Autodesk Inventor part; units mm, degrees
(part 2 of 2)
  line L515 (266.104, 188.0456) -> (266.9242, 187.2258) construction
  line L516 (266.9242, 187.2258) -> (266.9242, 186.2158) construction
  line L517 (266.9242, 186.2158) -> (266.9242, 185.2058) construction
  line L518 (266.9242, 185.2058) -> (266.104, 184.3855) construction
  line L519 (266.104, 184.3855) -> (265.094, 184.3855) construction
  spline S46 degree 3 poles (265.094, 168.3853) (264.084, 168.3853) (263.2642, 169.2052) (263.2642, 170.2152) (263.2642, 171.2255) (264.084, 172.0454) (265.094, 172.0454) (266.104, 172.0454) (266.9242, 171.2255) (266.9242, 170.2152) (266.9242, 169.2052) (266.104, 168.3853) (265.094, 168.3853) knots 0 0 0 0 1 1 1 2 2 2 3 3 3 4 4 4 4
  line L520 (265.094, 168.3853) -> (264.084, 168.3853) construction
  line L521 (264.084, 168.3853) -> (263.2642, 169.2052) construction
  line L522 (263.2642, 169.2052) -> (263.2642, 170.2152) construction
  line L523 (263.2642, 170.2152) -> (263.2642, 171.2255) construction
  line L524 (263.2642, 171.2255) -> (264.084, 172.0454) construction
  line L525 (264.084, 172.0454) -> (265.094, 172.0454) construction
  line L526 (265.094, 172.0454) -> (266.104, 172.0454) construction
  line L527 (266.104, 172.0454) -> (266.9242, 171.2255) construction
  line L528 (266.9242, 171.2255) -> (266.9242, 170.2152) construction
  line L529 (266.9242, 170.2152) -> (266.9242, 169.2052) construction
  line L530 (266.9242, 169.2052) -> (266.104, 168.3853) construction
  line L531 (266.104, 168.3853) -> (265.094, 168.3853) construction
  spline S47 degree 3 poles (265.0305, 152.3834) (264.0262, 152.3834) (263.2102, 153.2036) (263.2102, 154.2136) (263.2102, 155.2236) (264.0262, 156.0434) (265.0305, 156.0434) (266.0366, 156.0434) (266.8526, 155.2236) (266.8526, 154.2136) (266.8526, 153.2036) (266.0366, 152.3834) (265.0305, 152.3834) knots 0 0 0 0 1 1 1 2 2 2 3 3 3 4 4 4 4
  line L532 (265.0305, 152.3834) -> (264.0262, 152.3834) construction
  line L533 (264.0262, 152.3834) -> (263.2102, 153.2036) construction
  line L534 (263.2102, 153.2036) -> (263.2102, 154.2136) construction
  line L535 (263.2102, 154.2136) -> (263.2102, 155.2236) construction
  line L536 (263.2102, 155.2236) -> (264.0262, 156.0434) construction
  line L537 (264.0262, 156.0434) -> (265.0305, 156.0434) construction
  line L538 (265.0305, 156.0434) -> (266.0366, 156.0434) construction
  line L539 (266.0366, 156.0434) -> (266.8526, 155.2236) construction
  line L540 (266.8526, 155.2236) -> (266.8526, 154.2136) construction
  line L541 (266.8526, 154.2136) -> (266.8526, 153.2036) construction
  line L542 (266.8526, 153.2036) -> (266.0366, 152.3834) construction
  line L543 (266.0366, 152.3834) -> (265.0305, 152.3834) construction
  spline S48 degree 3 poles (265.0305, 136.3832) (264.0262, 136.3832) (263.2102, 137.203) (263.2102, 138.213) (263.2102, 139.2234) (264.0262, 140.0432) (265.0305, 140.0432) (266.0366, 140.0432) (266.8526, 139.2234) (266.8526, 138.213) (266.8526, 137.203) (266.0366, 136.3832) (265.0305, 136.3832) knots 0 0 0 0 1 1 1 2 2 2 3 3 3 4 4 4 4
  line L544 (265.0305, 136.3832) -> (264.0262, 136.3832) construction
  line L545 (264.0262, 136.3832) -> (263.2102, 137.203) construction
  line L546 (263.2102, 137.203) -> (263.2102, 138.213) construction
  line L547 (263.2102, 138.213) -> (263.2102, 139.2234) construction
  line L548 (263.2102, 139.2234) -> (264.0262, 140.0432) construction
  line L549 (264.0262, 140.0432) -> (265.0305, 140.0432) construction
  line L550 (265.0305, 140.0432) -> (266.0366, 140.0432) construction
  line L551 (266.0366, 140.0432) -> (266.8526, 139.2234) construction
  line L552 (266.8526, 139.2234) -> (266.8526, 138.213) construction
  line L553 (266.8526, 138.213) -> (266.8526, 137.203) construction
  line L554 (266.8526, 137.203) -> (266.0366, 136.3832) construction
  line L555 (266.0366, 136.3832) -> (265.0305, 136.3832) construction
  spline S49 degree 3 poles (264.901, 120.384) (263.9062, 120.384) (263.0987, 121.2039) (263.0987, 122.2142) (263.0987, 123.2228) (263.9062, 124.0427) (264.901, 124.0427) (265.8962, 124.0427) (266.7037, 123.2228) (266.7037, 122.2142) (266.7037, 121.2039) (265.8962, 120.384) (264.901, 120.384) knots 0 0 0 0 1 1 1 2 2 2 3 3 3 4 4 4 4
  line L556 (264.901, 120.384) -> (263.9062, 120.384) construction
  line L557 (263.9062, 120.384) -> (263.0987, 121.2039) construction
  line L558 (263.0987, 121.2039) -> (263.0987, 122.2142) construction
  line L559 (263.0987, 122.2142) -> (263.0987, 123.2228) construction
  line L560 (263.0987, 123.2228) -> (263.9062, 124.0427) construction
  line L561 (263.9062, 124.0427) -> (264.901, 124.0427) construction
  line L562 (264.901, 124.0427) -> (265.8962, 124.0427) construction
  line L563 (265.8962, 124.0427) -> (266.7037, 123.2228) construction
  line L564 (266.7037, 123.2228) -> (266.7037, 122.2142) construction
  line L565 (266.7037, 122.2142) -> (266.7037, 121.2039) construction
  line L566 (266.7037, 121.2039) -> (265.8962, 120.384) construction
  line L567 (265.8962, 120.384) -> (264.901, 120.384) construction
  spline S50 degree 3 poles (282.3572, 87.3704) (282.3572, 88.3808) (283.1771, 89.2007) (284.1871, 89.2007) (285.1974, 89.2007) (286.0173, 88.3808) (286.0173, 87.3704) (286.0173, 86.3604) (285.1974, 85.5406) (284.1871, 85.5406) (283.1771, 85.5406) (282.3572, 86.3604) (282.3572, 87.3704) knots 0 0 0 0 1 1 1 2 2 2 3 3 3 4 4 4 4
  line L568 (282.3572, 87.3704) -> (282.3572, 88.3808) construction
  line L569 (282.3572, 88.3808) -> (283.1771, 89.2007) construction
  line L570 (283.1771, 89.2007) -> (284.1871, 89.2007) construction
  line L571 (284.1871, 89.2007) -> (285.1974, 89.2007) construction
  line L572 (285.1974, 89.2007) -> (286.0173, 88.3808) construction
  line L573 (286.0173, 88.3808) -> (286.0173, 87.3704) construction
  line L574 (286.0173, 87.3704) -> (286.0173, 86.3604) construction
  line L575 (286.0173, 86.3604) -> (285.1974, 85.5406) construction
  line L576 (285.1974, 85.5406) -> (284.1871, 85.5406) construction
  line L577 (284.1871, 85.5406) -> (283.1771, 85.5406) construction
  line L578 (283.1771, 85.5406) -> (282.3572, 86.3604) construction
  line L579 (282.3572, 86.3604) -> (282.3572, 87.3704) construction
  spline S51 degree 3 poles (266.3566, 87.3704) (266.3566, 88.3808) (267.1768, 89.2007) (268.1868, 89.2007) (269.1968, 89.2007) (270.0167, 88.3808) (270.0167, 87.3704) (270.0167, 86.3604) (269.1968, 85.5406) (268.1868, 85.5406) (267.1768, 85.5406) (266.3566, 86.3604) (266.3566, 87.3704) knots 0 0 0 0 1 1 1 2 2 2 3 3 3 4 4 4 4
  line L580 (266.3566, 87.3704) -> (266.3566, 88.3808) construction
  line L581 (266.3566, 88.3808) -> (267.1768, 89.2007) construction
  line L582 (267.1768, 89.2007) -> (268.1868, 89.2007) construction
  line L583 (268.1868, 89.2007) -> (269.1968, 89.2007) construction
  line L584 (269.1968, 89.2007) -> (270.0167, 88.3808) construction
  line L585 (270.0167, 88.3808) -> (270.0167, 87.3704) construction
  line L586 (270.0167, 87.3704) -> (270.0167, 86.3604) construction
  line L587 (270.0167, 86.3604) -> (269.1968, 85.5406) construction
  line L588 (269.1968, 85.5406) -> (268.1868, 85.5406) construction
  line L589 (268.1868, 85.5406) -> (267.1768, 85.5406) construction
  line L590 (267.1768, 85.5406) -> (266.3566, 86.3604) construction
  line L591 (266.3566, 86.3604) -> (266.3566, 87.3704) construction
  spline S52 degree 3 poles (254.015, 87.4339) (254.015, 88.4387) (253.1952, 89.2543) (252.1852, 89.2543) (251.1748, 89.2543) (250.355, 88.4387) (250.355, 87.4339) (250.355, 86.4292) (251.1748, 85.6122) (252.1852, 85.6122) (253.1952, 85.6122) (254.015, 86.4292) (254.015, 87.4339) knots 0 0 0 0 1 1 1 2 2 2 3 3 3 4 4 4 4
  line L592 (254.015, 87.4339) -> (254.015, 88.4387) construction
  line L593 (254.015, 88.4387) -> (253.1952, 89.2543) construction
  line L594 (253.1952, 89.2543) -> (252.1852, 89.2543) construction
  line L595 (252.1852, 89.2543) -> (251.1748, 89.2543) construction
  line L596 (251.1748, 89.2543) -> (250.355, 88.4387) construction
  line L597 (250.355, 88.4387) -> (250.355, 87.4339) construction
  line L598 (250.355, 87.4339) -> (250.355, 86.4292) construction
  line L599 (250.355, 86.4292) -> (251.1748, 85.6122) construction
  line L600 (251.1748, 85.6122) -> (252.1852, 85.6122) construction
  line L601 (252.1852, 85.6122) -> (253.1952, 85.6122) construction
  line L602 (253.1952, 85.6122) -> (254.015, 86.4292) construction
  line L603 (254.015, 86.4292) -> (254.015, 87.4339) construction
  spline S53 degree 3 poles (234.3547, 87.4339) (234.3547, 88.4387) (235.1746, 89.2543) (236.1846, 89.2543) (237.1946, 89.2543) (238.0148, 88.4387) (238.0148, 87.4339) (238.0148, 86.4292) (237.1946, 85.6122) (236.1846, 85.6122) (235.1746, 85.6122) (234.3547, 86.4292) (234.3547, 87.4339) knots 0 0 0 0 1 1 1 2 2 2 3 3 3 4 4 4 4
  line L604 (234.3547, 87.4339) -> (234.3547, 88.4387) construction
  line L605 (234.3547, 88.4387) -> (235.1746, 89.2543) construction
  line L606 (235.1746, 89.2543) -> (236.1846, 89.2543) construction
  line L607 (236.1846, 89.2543) -> (237.1946, 89.2543) construction
  line L608 (237.1946, 89.2543) -> (238.0148, 88.4387) construction
  line L609 (238.0148, 88.4387) -> (238.0148, 87.4339) construction
  line L610 (238.0148, 87.4339) -> (238.0148, 86.4292) construction
  line L611 (238.0148, 86.4292) -> (237.1946, 85.6122) construction
  line L612 (237.1946, 85.6122) -> (236.1846, 85.6122) construction
  line L613 (236.1846, 85.6122) -> (235.1746, 85.6122) construction
  line L614 (235.1746, 85.6122) -> (234.3547, 86.4292) construction
  line L615 (234.3547, 86.4292) -> (234.3547, 87.4339) construction
  spline S54 degree 3 poles (218.3542, 87.5634) (218.3542, 88.5586) (219.1754, 89.3661) (220.1844, 89.3661) (221.1944, 89.3661) (222.0142, 88.5586) (222.0142, 87.5634) (222.0142, 86.5686) (221.1944, 85.7611) (220.1844, 85.7611) (219.1754, 85.7611) (218.3542, 86.5686) (218.3542, 87.5634) knots 0 0 0 0 1 1 1 2 2 2 3 3 3 4 4 4 4
  line L616 (218.3542, 87.5634) -> (218.3542, 88.5586) construction
  line L617 (218.3542, 88.5586) -> (219.1754, 89.3661) construction
  line L618 (219.1754, 89.3661) -> (220.1844, 89.3661) construction
  line L619 (220.1844, 89.3661) -> (221.1944, 89.3661) construction
  line L620 (221.1944, 89.3661) -> (222.0142, 88.5586) construction
  line L621 (222.0142, 88.5586) -> (222.0142, 87.5634) construction
  line L622 (222.0142, 87.5634) -> (222.0142, 86.5686) construction
  line L623 (222.0142, 86.5686) -> (221.1944, 85.7611) construction
  line L624 (221.1944, 85.7611) -> (220.1844, 85.7611) construction
  line L625 (220.1844, 85.7611) -> (219.1754, 85.7611) construction
  line L626 (219.1754, 85.7611) -> (218.3542, 86.5686) construction
  line L627 (218.3542, 86.5686) -> (218.3542, 87.5634) construction
  spline S55 degree 3 poles (282.3569, 7.3714) (282.3569, 8.3814) (283.1771, 9.2012) (284.1871, 9.2012) (285.1971, 9.2012) (286.0169, 8.3814) (286.0169, 7.3714) (286.0169, 6.3614) (285.1971, 5.5412) (284.1871, 5.5412) (283.1771, 5.5412) (282.3569, 6.3614) (282.3569, 7.3714) knots 0 0 0 0 1 1 1 2 2 2 3 3 3 4 4 4 4
  line L628 (282.3569, 7.3714) -> (282.3569, 8.3814) construction
  line L629 (282.3569, 8.3814) -> (283.1771, 9.2012) construction
  line L630 (283.1771, 9.2012) -> (284.1871, 9.2012) construction
  line L631 (284.1871, 9.2012) -> (285.1971, 9.2012) construction
  line L632 (285.1971, 9.2012) -> (286.0169, 8.3814) construction
  line L633 (286.0169, 8.3814) -> (286.0169, 7.3714) construction
  line L634 (286.0169, 7.3714) -> (286.0169, 6.3614) construction
  line L635 (286.0169, 6.3614) -> (285.1971, 5.5412) construction
  line L636 (285.1971, 5.5412) -> (284.1871, 5.5412) construction
  line L637 (284.1871, 5.5412) -> (283.1771, 5.5412) construction
  line L638 (283.1771, 5.5412) -> (282.3569, 6.3614) construction
  line L639 (282.3569, 6.3614) -> (282.3569, 7.3714) construction
  spline S56 degree 3 poles (266.3566, 7.3714) (266.3566, 8.3814) (267.1765, 9.2012) (268.1865, 9.2012) (269.1968, 9.2012) (270.0167, 8.3814) (270.0167, 7.3714) (270.0167, 6.3614) (269.1968, 5.5412) (268.1865, 5.5412) (267.1765, 5.5412) (266.3566, 6.3614) (266.3566, 7.3714) knots 0 0 0 0 1 1 1 2 2 2 3 3 3 4 4 4 4
  line L640 (266.3566, 7.3714) -> (266.3566, 8.3814) construction
  line L641 (266.3566, 8.3814) -> (267.1765, 9.2012) construction
  line L642 (267.1765, 9.2012) -> (268.1865, 9.2012) construction
  line L643 (268.1865, 9.2012) -> (269.1968, 9.2012) construction
  line L644 (269.1968, 9.2012) -> (270.0167, 8.3814) construction
  line L645 (270.0167, 8.3814) -> (270.0167, 7.3714) construction
  line L646 (270.0167, 7.3714) -> (270.0167, 6.3614) construction
  line L647 (270.0167, 6.3614) -> (269.1968, 5.5412) construction
  line L648 (269.1968, 5.5412) -> (268.1865, 5.5412) construction
  line L649 (268.1865, 5.5412) -> (267.1765, 5.5412) construction
  line L650 (267.1765, 5.5412) -> (266.3566, 6.3614) construction
  line L651 (266.3566, 6.3614) -> (266.3566, 7.3714) construction
  spline S57 degree 3 poles (250.3546, 7.4349) (250.3546, 8.4392) (251.1748, 9.2552) (252.1848, 9.2552) (253.1948, 9.2552) (254.0147, 8.4392) (254.0147, 7.4349) (254.0147, 6.4288) (253.1948, 5.6128) (252.1848, 5.6128) (251.1748, 5.6128) (250.3546, 6.4288) (250.3546, 7.4349) knots 0 0 0 0 1 1 1 2 2 2 3 3 3 4 4 4 4
  line L652 (250.3546, 7.4349) -> (250.3546, 8.4392) construction
  line L653 (250.3546, 8.4392) -> (251.1748, 9.2552) construction
  line L654 (251.1748, 9.2552) -> (252.1848, 9.2552) construction
  line L655 (252.1848, 9.2552) -> (253.1948, 9.2552) construction
  line L656 (253.1948, 9.2552) -> (254.0147, 8.4392) construction
  line L657 (254.0147, 8.4392) -> (254.0147, 7.4349) construction
  line L658 (254.0147, 7.4349) -> (254.0147, 6.4288) construction
  line L659 (254.0147, 6.4288) -> (253.1948, 5.6128) construction
  line L660 (253.1948, 5.6128) -> (252.1848, 5.6128) construction
  line L661 (252.1848, 5.6128) -> (251.1748, 5.6128) construction
  line L662 (251.1748, 5.6128) -> (250.3546, 6.4288) construction
  line L663 (250.3546, 6.4288) -> (250.3546, 7.4349) construction
  spline S58 degree 3 poles (234.3544, 7.4349) (234.3544, 8.4392) (235.1743, 9.2552) (236.1843, 9.2552) (237.1946, 9.2552) (238.0145, 8.4392) (238.0145, 7.4349) (238.0145, 6.4288) (237.1946, 5.6128) (236.1843, 5.6128) (235.1743, 5.6128) (234.3544, 6.4288) (234.3544, 7.4349) knots 0 0 0 0 1 1 1 2 2 2 3 3 3 4 4 4 4
  line L664 (234.3544, 7.4349) -> (234.3544, 8.4392) construction
  line L665 (234.3544, 8.4392) -> (235.1743, 9.2552) construction
  line L666 (235.1743, 9.2552) -> (236.1843, 9.2552) construction
  line L667 (236.1843, 9.2552) -> (237.1946, 9.2552) construction
  line L668 (237.1946, 9.2552) -> (238.0145, 8.4392) construction
  line L669 (238.0145, 8.4392) -> (238.0145, 7.4349) construction
  line L670 (238.0145, 7.4349) -> (238.0145, 6.4288) construction
  line L671 (238.0145, 6.4288) -> (237.1946, 5.6128) construction
  line L672 (237.1946, 5.6128) -> (236.1843, 5.6128) construction
  line L673 (236.1843, 5.6128) -> (235.1743, 5.6128) construction
  line L674 (235.1743, 5.6128) -> (234.3544, 6.4288) construction
  line L675 (234.3544, 6.4288) -> (234.3544, 7.4349) construction
  spline S59 degree 3 poles (218.3552, 7.5643) (218.3552, 8.5592) (219.1751, 9.3667) (220.1854, 9.3667) (221.194, 9.3667) (222.0139, 8.5592) (222.0139, 7.5643) (222.0139, 6.5692) (221.194, 5.7617) (220.1854, 5.7617) (219.1751, 5.7617) (218.3552, 6.5692) (218.3552, 7.5643) knots 0 0 0 0 1 1 1 2 2 2 3 3 3 4 4 4 4
  line L676 (218.3552, 7.5643) -> (218.3552, 8.5592) construction
  line L677 (218.3552, 8.5592) -> (219.1751, 9.3667) construction
  line L678 (219.1751, 9.3667) -> (220.1854, 9.3667) construction
  line L679 (220.1854, 9.3667) -> (221.194, 9.3667) construction
  line L680 (221.194, 9.3667) -> (222.0139, 8.5592) construction
  line L681 (222.0139, 8.5592) -> (222.0139, 7.5643) construction
  line L682 (222.0139, 7.5643) -> (222.0139, 6.5692) construction
  line L683 (222.0139, 6.5692) -> (221.194, 5.7617) construction
  line L684 (221.194, 5.7617) -> (220.1854, 5.7617) construction
  line L685 (220.1854, 5.7617) -> (219.1751, 5.7617) construction
  line L686 (219.1751, 5.7617) -> (218.3552, 6.5692) construction
  line L687 (218.3552, 6.5692) -> (218.3552, 7.5643) construction
  point P0 (0, 0)
  constraints: 8 end point, 124 other
extrude "Extrusion1" add sketch "Sketch1" along normal blind 2.032
sketch "Sketch2" plane through (0, 0, 2.032) normal (0, 0, 1) x (1, 0, 0)
  circle A0 centre (12.6982, 174.6292) radius 3.212
  circle A1 centre (12.6982, 28.5838) radius 3.212
  circle A2 centre (327.3038, 174.6292) radius 3.212
  circle A3 centre (327.2724, 28.5838) radius 3.212
  point P0 (0, 0)
  constraints: 4 centre point
extrude "Extrusion2" cut sketch "Sketch2" against normal blind 17.4625
body "Solid1"
